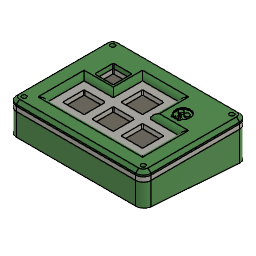
Hackpad (Autodesk Fusion 360 design; units mm, degrees)
Autodesk Fusion 360 part; units mm, degrees
sketch "Main" plane through (0, 0, 0) normal (0, 0, 1) x (1, 0, 0)
  line L0 (33.9, -23.9) -> (-33.9, -23.9)
  line L1 (-33.9, -23.9) -> (-33.9, 23.9)
  line L2 (-33.9, 23.9) -> (33.9, 23.9)
  line L3 (33.9, 23.9) -> (33.9, -23.9)
  line L4 (33.9, -23.9) -> (-33.9, 23.9) construction
  line L5 (-33.9, -23.9) -> (33.9, 23.9) construction
  line L6 (43.9, -33.9) -> (-43.9, -33.9)
  line L7 (-43.9, -33.9) -> (-43.9, 33.9)
  line L8 (-43.9, 33.9) -> (43.9, 33.9)
  line L9 (43.9, 33.9) -> (43.9, -33.9)
  circle A0 centre (-38.9, 28.9) radius 1.45
  circle A1 centre (-38.9, -28.9) radius 1.45
  circle A2 centre (38.9, 28.9) radius 1.45
  circle A3 centre (38.9, -28.9) radius 1.45
  arc A4 (-12.125, -3.025) -> (-12.625, -2.525) centre (-12.625, -3.025) ccw
  arc A5 (-12.625, -16.525) -> (-12.125, -16.025) centre (-12.625, -16.025) ccw
  line L10 (-25.625, -16.525) -> (-12.625, -16.525)
  arc A6 (-26.125, -16.025) -> (-25.625, -16.525) centre (-25.625, -16.025) ccw
  line L11 (-26.125, -3.025) -> (-26.125, -16.025)
  arc A7 (-25.625, -2.525) -> (-26.125, -3.025) centre (-25.625, -3.025) ccw
  line L12 (-25.625, -2.525) -> (-12.625, -2.525)
  line L13 (-6.575, -16.525) -> (6.425, -16.525)
  arc A8 (6.425, -16.525) -> (6.925, -16.025) centre (6.425, -16.025) ccw
  line L14 (6.925, -3.025) -> (6.925, -16.025)
  arc A9 (6.925, -3.025) -> (6.425, -2.525) centre (6.425, -3.025) ccw
  line L15 (-6.575, -2.525) -> (6.425, -2.525)
  arc A10 (-6.575, -2.525) -> (-7.075, -3.025) centre (-6.575, -3.025) ccw
  arc A11 (-7.075, -16.025) -> (-6.575, -16.525) centre (-6.575, -16.025) ccw
  line L16 (-7.075, -3.025) -> (-7.075, -16.025)
  line L17 (12.475, -16.525) -> (25.475, -16.525)
  arc A12 (25.475, -16.525) -> (25.975, -16.025) centre (25.475, -16.025) ccw
  line L18 (25.975, -3.025) -> (25.975, -16.025)
  arc A13 (25.975, -3.025) -> (25.475, -2.525) centre (25.475, -3.025) ccw
  line L19 (12.475, -2.525) -> (25.475, -2.525)
  arc A14 (12.475, -2.525) -> (11.975, -3.025) centre (12.475, -3.025) ccw
  arc A15 (11.975, -16.025) -> (12.475, -16.525) centre (12.475, -16.025) ccw
  arc A16 (6.425, 2.525) -> (6.925, 3.025) centre (6.425, 3.025) ccw
  arc A17 (-7.075, 3.025) -> (-6.575, 2.525) centre (-6.575, 3.025) ccw
  line L20 (-7.075, 16.025) -> (-7.075, 3.025)
  arc A18 (-6.575, 16.525) -> (-7.075, 16.025) centre (-6.575, 16.025) ccw
  line L21 (-6.575, 16.525) -> (6.425, 16.525)
  arc A19 (6.925, 16.025) -> (6.425, 16.525) centre (6.425, 16.025) ccw
  line L22 (6.925, 16.025) -> (6.925, 3.025)
  line L23 (-6.575, 2.525) -> (6.425, 2.525)
  line L24 (-31.175, 21.575) -> (31.025, 21.575)
  line L25 (-31.175, 21.575) -> (-31.175, -21.575)
  line L26 (-31.175, -21.575) -> (31.025, -21.575)
  line L27 (31.025, 21.575) -> (31.025, -21.575)
  line L28 (11.975, -3.025) -> (11.975, -16.025)
  line L29 (-12.125, -3.025) -> (-12.125, -16.025)
  line L30 (-12.125, 21.575) -> (-12.125, 2.525)
  line L31 (-31.175, 2.525) -> (-12.125, 2.525)
  line L32 (11.975, 2.525) -> (31.025, 2.525)
  line L33 (11.975, 21.575) -> (11.975, 2.525)
  line L34 (-16.95, 6.85) -> (-28.15, 6.85)
  line L35 (-28.65, 7.35) -> (-28.65, 18.55)
  line L36 (-28.15, 19.05) -> (-16.95, 19.05)
  line L37 (-16.45, 18.55) -> (-16.45, 7.35)
  line L38 (-16.45, 6.85) -> (-28.65, 19.05) construction
  line L39 (-28.65, 6.85) -> (-16.45, 19.05) construction
  arc A20 (-28.15, 19.05) -> (-28.65, 18.55) centre (-28.15, 18.55) ccw
  arc A21 (-16.45, 18.55) -> (-16.95, 19.05) centre (-16.95, 18.55) ccw
  arc A22 (-28.65, 7.35) -> (-28.15, 6.85) centre (-28.15, 7.35) ccw
  arc A23 (-16.95, 6.85) -> (-16.45, 7.35) centre (-16.95, 7.35) ccw
  line L40 (9.45, 0) -> (-9.6, 0)
  line L41 (-9.6, 0) -> (-9.6, 19.05)
  line L42 (-9.6, 19.05) -> (9.45, 19.05)
  line L43 (9.45, 19.05) -> (9.45, 0)
  line L44 (9.45, 0) -> (-9.6, 19.05) construction
  line L45 (-9.6, 0) -> (9.45, 19.05) construction
  line L46 (-9.6, -19.05) -> (-28.65, -19.05)
  line L47 (-28.65, -19.05) -> (-28.65, 0)
  line L48 (-28.65, 0) -> (-9.6, 0)
  line L49 (-9.6, 0) -> (-9.6, -19.05)
  line L50 (0, 23.9) -> (0, -33.9) construction
  arc A24 (16.95, 19.05) -> (16.45, 18.55) centre (16.95, 18.55) ccw
  line L51 (16.45, 18.55) -> (16.45, 7.35)
  arc A25 (16.45, 7.35) -> (16.95, 6.85) centre (16.95, 7.35) ccw
  line L52 (16.95, 6.85) -> (28.15, 6.85)
  arc A26 (28.15, 6.85) -> (28.65, 7.35) centre (28.15, 7.35) ccw
  line L53 (28.65, 7.35) -> (28.65, 18.55)
  arc A27 (28.65, 18.55) -> (28.15, 19.05) centre (28.15, 18.55) ccw
  line L54 (28.15, 19.05) -> (16.95, 19.05)
  spline S0 degree 3 poles (22.2716, 17.9984) (22.4772, 17.9984) (22.6828, 17.9984) (22.8884, 17.9984) knots 0 0 0 0 1 1 1 1
  spline S1 degree 3 poles (22.8884, 17.9984) (22.9326, 17.9794) (23.084, 17.9645) (23.1108, 17.9887) knots 0 0 0 0 1 1 1 1
  spline S2 degree 3 poles (23.1108, 17.9887) (23.1434, 17.9593) (23.3545, 17.9395) (23.4085, 17.9401) knots 0 0 0 0 1 1 1 1
  spline S3 degree 3 poles (23.4085, 17.9401) (23.4406, 17.9405) (23.4795, 17.918) (23.5093, 17.9135) knots 0 0 0 0 1 1 1 1
  spline S4 degree 3 poles (23.5093, 17.9135) (23.5998, 17.8996) (23.701, 17.8877) (23.795, 17.8676) knots 0 0 0 0 1 1 1 1
  spline S5 degree 3 poles (23.795, 17.8676) (23.8778, 17.85) (23.9581, 17.8109) (24.0419, 17.7948) knots 0 0 0 0 1 1 1 1
  spline S6 degree 3 poles (24.0419, 17.7948) (24.058, 17.7918) (24.0679, 17.7758) (24.0836, 17.7722) knots 0 0 0 0 1 1 1 1
  spline S7 degree 3 poles (24.0836, 17.7722) (24.2356, 17.7361) (24.382, 17.6718) (24.5308, 17.6218) knots 0 0 0 0 1 1 1 1
  spline S8 degree 3 poles (24.5308, 17.6218) (24.5703, 17.6085) (24.6731, 17.5303) (24.6983, 17.5523) knots 0 0 0 0 1 1 1 1
  spline S9 degree 3 poles (24.6983, 17.5523) (24.7382, 17.498) (24.8225, 17.4853) (24.8785, 17.4541) knots 0 0 0 0 1 1 1 1
  spline S10 degree 3 poles (24.8785, 17.4541) (24.9607, 17.4083) (25.0549, 17.3585) (25.1345, 17.3031) knots 0 0 0 0 1 1 1 1
  spline S11 degree 3 poles (25.1345, 17.3031) (25.4383, 17.0916) (25.751, 16.8719) (25.9987, 16.579) knots 0 0 0 0 1 1 1 1
  spline S12 degree 3 poles (25.9987, 16.579) (26.1039, 16.4548) (26.216, 16.3169) (26.3112, 16.1875) knots 0 0 0 0 1 1 1 1
  spline S13 degree 3 poles (26.3112, 16.1875) (26.3854, 16.0869) (26.442, 15.9672) (26.5144, 15.8634) knots 0 0 0 0 1 1 1 1
  spline S14 degree 3 poles (26.5144, 15.8634) (26.567, 15.7884) (26.6319, 15.5622) (26.6964, 15.5146) knots 0 0 0 0 1 1 1 1
  spline S15 degree 3 poles (26.6964, 15.5146) (26.6815, 15.4925) (26.715, 15.4554) (26.7295, 15.4265) knots 0 0 0 0 1 1 1 1
  spline S16 degree 3 poles (26.7295, 15.4265) (26.751, 15.3836) (26.8186, 15.2094) (26.8289, 15.1655) knots 0 0 0 0 1 1 1 1
  spline S17 degree 3 poles (26.8289, 15.1655) (26.8895, 14.9066) (27.0063, 14.6397) (27.0157, 14.3835) knots 0 0 0 0 1 1 1 1
  spline S18 degree 3 poles (27.0157, 14.3835) (27.0165, 14.3601) (27.0395, 14.3357) (27.0419, 14.3136) knots 0 0 0 0 1 1 1 1
  spline S19 degree 3 poles (27.0419, 14.3136) (27.0494, 14.2414) (27.05, 14.1612) (27.0554, 14.0957) knots 0 0 0 0 1 1 1 1
  spline S20 degree 3 poles (27.0554, 14.0957) (27.0579, 14.0646) (27.0812, 14.0261) (27.0845, 13.9961) knots 0 0 0 0 1 1 1 1
  spline S21 degree 3 poles (27.0845, 13.9961) (27.0893, 13.9552) (27.0613, 13.9424) (27.0935, 13.9072) knots 0 0 0 0 1 1 1 1
  spline S22 degree 3 poles (27.0935, 13.9072) (27.0431, 13.8523) (27.1145, 13.7201) (27.1062, 13.6592) knots 0 0 0 0 1 1 1 1
  spline S23 degree 3 poles (27.1062, 13.6592) (27.0869, 13.5175) (27.0736, 13.1639) (27.0945, 13.0242) knots 0 0 0 0 1 1 1 1
  spline S24 degree 3 poles (27.0945, 13.0242) (27.0996, 12.9893) (27.1085, 12.9617) (27.1072, 12.925) knots 0 0 0 0 1 1 1 1
  spline S25 degree 3 poles (27.1072, 12.925) (27.106, 12.8912) (27.0897, 12.8686) (27.0883, 12.8357) knots 0 0 0 0 1 1 1 1
  spline S26 degree 3 poles (27.0883, 12.8357) (27.0855, 12.7708) (27.0597, 12.5648) (27.0935, 12.5281) knots 0 0 0 0 1 1 1 1
  spline S27 degree 3 poles (27.0935, 12.5281) (27.0613, 12.4858) (27.0871, 12.4636) (27.0861, 12.4189) knots 0 0 0 0 1 1 1 1
  spline S28 degree 3 poles (27.0861, 12.4189) (27.0849, 12.361) (27.0294, 12.2788) (27.0734, 12.2304) knots 0 0 0 0 1 1 1 1
  spline S29 degree 3 poles (27.0734, 12.2304) (27.0415, 12.1953) (27.0439, 12.1016) (27.0444, 12.0518) knots 0 0 0 0 1 1 1 1
  spline S30 degree 3 poles (27.0444, 12.0518) (27.0448, 12.0125) (27.0167, 11.9735) (27.0157, 11.9328) knots 0 0 0 0 1 1 1 1
  spline S31 degree 3 poles (27.0157, 11.9328) (27.0141, 11.8609) (27.0046, 11.771) (26.9887, 11.6964) knots 0 0 0 0 1 1 1 1
  spline S32 degree 3 poles (26.9887, 11.6964) (26.9837, 11.674) (26.9623, 11.6478) (26.9577, 11.6234) knots 0 0 0 0 1 1 1 1
  spline S33 degree 3 poles (26.9577, 11.6234) (26.9111, 11.3785) (26.8113, 11.1164) (26.6883, 10.9025) knots 0 0 0 0 1 1 1 1
  spline S34 degree 3 poles (26.6883, 10.9025) (26.5359, 10.638) (26.217, 10.3324) (25.959, 10.1774) knots 0 0 0 0 1 1 1 1
  spline S35 degree 3 poles (25.959, 10.1774) (25.8709, 10.1246) (25.7862, 10.0796) (25.6921, 10.0333) knots 0 0 0 0 1 1 1 1
  spline S36 degree 3 poles (25.6921, 10.0333) (25.6417, 10.0087) (25.5661, 10.0024) (25.5318, 9.9544) knots 0 0 0 0 1 1 1 1
  spline S37 degree 3 poles (25.5318, 9.9544) (25.527, 9.9575) (25.529, 9.9669) (25.5218, 9.968) knots 0 0 0 0 1 1 1 1
  spline S38 degree 3 poles (25.5218, 9.968) (25.5197, 9.9684) (25.5038, 9.9522) (25.5004, 9.95) knots 0 0 0 0 1 1 1 1
  spline S39 degree 3 poles (25.5004, 9.95) (25.4738, 9.9327) (25.4397, 9.9355) (25.4127, 9.9236) knots 0 0 0 0 1 1 1 1
  spline S40 degree 3 poles (25.4127, 9.9236) (25.3724, 9.8541) (25.4006, 9.5845) (25.4006, 9.492) knots 0 0 0 0 1 1 1 1
  spline S41 degree 3 poles (25.4006, 9.492) (25.4006, 9.1666) (25.451, 8.6266) (25.3405, 8.3498) knots 0 0 0 0 1 1 1 1
  spline S42 degree 3 poles (25.3405, 8.3498) (25.27, 8.1732) (25.1008, 8.0081) (24.9275, 7.9172) knots 0 0 0 0 1 1 1 1
  spline S43 degree 3 poles (24.9275, 7.9172) (24.8791, 7.892) (24.7993, 7.8638) (24.7475, 7.8531) knots 0 0 0 0 1 1 1 1
  spline S44 degree 3 poles (24.7475, 7.8531) (24.7194, 7.8471) (24.7027, 7.859) (24.6749, 7.8416) knots 0 0 0 0 1 1 1 1
  spline S45 degree 3 poles (24.6749, 7.8416) (24.5949, 7.8416) (24.5148, 7.8416) (24.4346, 7.8416) knots 0 0 0 0 1 1 1 1
  spline S46 degree 3 poles (24.4346, 7.8416) (24.4056, 7.861) (24.3828, 7.8473) (24.3528, 7.8559) knots 0 0 0 0 1 1 1 1
  spline S47 degree 3 poles (24.3528, 7.8559) (24.2677, 7.8803) (24.1572, 7.9281) (24.0824, 7.9737) knots 0 0 0 0 1 1 1 1
  spline S48 degree 3 poles (24.0824, 7.9737) (24.0443, 7.997) (24.0078, 8.0718) (23.9641, 8.0652) knots 0 0 0 0 1 1 1 1
  spline S49 degree 3 poles (23.9641, 8.0652) (23.9417, 8.1222) (23.8843, 8.1631) (23.8448, 8.2111) knots 0 0 0 0 1 1 1 1
  spline S50 degree 3 poles (23.8448, 8.2111) (23.8181, 8.2434) (23.7587, 8.3702) (23.7484, 8.4123) knots 0 0 0 0 1 1 1 1
  spline S51 degree 3 poles (23.7484, 8.4123) (23.6914, 8.6421) (23.7095, 8.9066) (23.7095, 9.1546) knots 0 0 0 0 1 1 1 1
  spline S52 degree 3 poles (23.7095, 9.1546) (23.7095, 9.2572) (23.7095, 9.3596) (23.7095, 9.4622) knots 0 0 0 0 1 1 1 1
  spline S53 degree 3 poles (23.7095, 9.4622) (23.7095, 9.5015) (23.723, 9.5543) (23.6863, 9.5763) knots 0 0 0 0 1 1 1 1
  spline S54 degree 3 poles (23.6863, 9.5763) (23.6464, 9.573) (23.6369, 9.573) (23.597, 9.5763) knots 0 0 0 0 1 1 1 1
  spline S55 degree 3 poles (23.597, 9.5763) (23.544, 9.5698) (23.4912, 9.563) (23.4382, 9.5565) knots 0 0 0 0 1 1 1 1
  spline S56 degree 3 poles (23.4382, 9.5565) (23.4613, 9.4164) (23.4418, 9.2574) (23.4418, 9.115) knots 0 0 0 0 1 1 1 1
  spline S57 degree 3 poles (23.4418, 9.115) (23.4418, 8.7514) (23.4509, 8.4607) (23.2527, 8.1635) knots 0 0 0 0 1 1 1 1
  spline S58 degree 3 poles (23.2527, 8.1635) (23.2092, 8.0984) (23.0898, 7.992) (23.0221, 7.9555) knots 0 0 0 0 1 1 1 1
  spline S59 degree 3 poles (23.0221, 7.9555) (22.9693, 7.9267) (22.8959, 7.9128) (22.8529, 7.8708) knots 0 0 0 0 1 1 1 1
  spline S60 degree 3 poles (22.8529, 7.8708) (22.8306, 7.8878) (22.7316, 7.8624) (22.7003, 7.8416) knots 0 0 0 0 1 1 1 1
  spline S61 degree 3 poles (22.7003, 7.8416) (22.6201, 7.8416) (22.5399, 7.8416) (22.4597, 7.8416) knots 0 0 0 0 1 1 1 1
  spline S62 degree 3 poles (22.4597, 7.8416) (22.4151, 7.8718) (22.3671, 7.8596) (22.3189, 7.8761) knots 0 0 0 0 1 1 1 1
  spline S63 degree 3 poles (22.3189, 7.8761) (22.2298, 7.9067) (22.0371, 8.0047) (21.9744, 8.0823) knots 0 0 0 0 1 1 1 1
  spline S64 degree 3 poles (21.9744, 8.0823) (21.7025, 8.4184) (21.7182, 8.6715) (21.7182, 9.105) knots 0 0 0 0 1 1 1 1
  spline S65 degree 3 poles (21.7182, 9.105) (21.7182, 9.2505) (21.6983, 9.4132) (21.7218, 9.5565) knots 0 0 0 0 1 1 1 1
  spline S66 degree 3 poles (21.7218, 9.5565) (21.6688, 9.563) (21.616, 9.5698) (21.563, 9.5763) knots 0 0 0 0 1 1 1 1
  spline S67 degree 3 poles (21.563, 9.5763) (21.5231, 9.573) (21.5136, 9.573) (21.4737, 9.5763) knots 0 0 0 0 1 1 1 1
  spline S68 degree 3 poles (21.4737, 9.5763) (21.4275, 9.5485) (21.4505, 9.4237) (21.4505, 9.3729) knots 0 0 0 0 1 1 1 1
  spline S69 degree 3 poles (21.4505, 9.3729) (21.4505, 9.1745) (21.4505, 8.9761) (21.4505, 8.7776) knots 0 0 0 0 1 1 1 1
  spline S70 degree 3 poles (21.4505, 8.7776) (21.4505, 8.6284) (21.4432, 8.4766) (21.3824, 8.3434) knots 0 0 0 0 1 1 1 1
  spline S71 degree 3 poles (21.3824, 8.3434) (21.3654, 8.3059) (21.3412, 8.2404) (21.3154, 8.2111) knots 0 0 0 0 1 1 1 1
  spline S72 degree 3 poles (21.3154, 8.2111) (21.3017, 8.1954) (21.2384, 8.1488) (21.2368, 8.1273) knots 0 0 0 0 1 1 1 1
  spline S73 degree 3 poles (21.2368, 8.1273) (21.2362, 8.122) (21.2427, 8.1182) (21.2435, 8.1129) knots 0 0 0 0 1 1 1 1
  spline S74 degree 3 poles (21.2435, 8.1129) (21.1782, 8.088) (21.1368, 8.012) (21.0776, 7.9734) knots 0 0 0 0 1 1 1 1
  spline S75 degree 3 poles (21.0776, 7.9734) (21.0165, 7.9335) (20.8766, 7.8688) (20.8072, 7.8559) knots 0 0 0 0 1 1 1 1
  spline S76 degree 3 poles (20.8072, 7.8559) (20.776, 7.8501) (20.7538, 7.8612) (20.7252, 7.8416) knots 0 0 0 0 1 1 1 1
  spline S77 degree 3 poles (20.7252, 7.8416) (20.645, 7.8416) (20.5651, 7.8416) (20.4849, 7.8416) knots 0 0 0 0 1 1 1 1
  spline S78 degree 3 poles (20.4849, 7.8416) (20.4399, 7.8684) (20.3827, 7.8622) (20.3345, 7.8779) knots 0 0 0 0 1 1 1 1
  spline S79 degree 3 poles (20.3345, 7.8779) (20.1944, 7.9229) (20.0555, 8.0232) (19.9576, 8.1325) knots 0 0 0 0 1 1 1 1
  spline S80 degree 3 poles (19.9576, 8.1325) (19.8876, 8.2107) (19.8301, 8.3172) (19.7943, 8.4109) knots 0 0 0 0 1 1 1 1
  spline S81 degree 3 poles (19.7943, 8.4109) (19.7469, 8.5349) (19.7594, 8.6879) (19.7594, 8.8272) knots 0 0 0 0 1 1 1 1
  spline S82 degree 3 poles (19.7594, 8.8272) (19.7594, 9.0654) (19.7594, 9.3035) (19.7594, 9.5416) knots 0 0 0 0 1 1 1 1
  spline S83 degree 3 poles (19.7594, 9.5416) (19.7594, 9.6559) (19.7862, 9.8101) (19.7523, 9.9186) knots 0 0 0 0 1 1 1 1
  spline S84 degree 3 poles (19.7523, 9.9186) (19.7288, 9.9353) (19.6453, 9.9665) (19.6282, 9.9544) knots 0 0 0 0 1 1 1 1
  spline S85 degree 3 poles (19.6282, 9.9544) (19.5953, 9.9986) (19.3961, 10.0689) (19.3391, 10.098) knots 0 0 0 0 1 1 1 1
  spline S86 degree 3 poles (19.3391, 10.098) (19.1699, 10.1849) (19.0292, 10.309) (18.8754, 10.4217) knots 0 0 0 0 1 1 1 1
  spline S87 degree 3 poles (18.8754, 10.4217) (18.748, 10.5151) (18.5432, 10.7767) (18.4688, 10.9102) knots 0 0 0 0 1 1 1 1
  spline S88 degree 3 poles (18.4688, 10.9102) (18.4336, 10.9729) (18.4073, 11.0938) (18.3447, 11.139) knots 0 0 0 0 1 1 1 1
  spline S89 degree 3 poles (18.3447, 11.139) (18.365, 11.1696) (18.3027, 11.2454) (18.2914, 11.2896) knots 0 0 0 0 1 1 1 1
  spline S90 degree 3 poles (18.2914, 11.2896) (18.2682, 11.3799) (18.214, 11.4984) (18.2013, 11.5873) knots 0 0 0 0 1 1 1 1
  spline S91 degree 3 poles (18.2013, 11.5873) (18.1925, 11.647) (18.1798, 11.7504) (18.1463, 11.7939) knots 0 0 0 0 1 1 1 1
  spline S92 degree 3 poles (18.1463, 11.7939) (18.1781, 11.8292) (18.1348, 11.8687) (18.1354, 11.9129) knots 0 0 0 0 1 1 1 1
  spline S93 degree 3 poles (18.1354, 11.9129) (18.136, 11.9663) (18.115, 12.1993) (18.0864, 12.2304) knots 0 0 0 0 1 1 1 1
  spline S94 degree 3 poles (18.0864, 12.2304) (18.1277, 12.2755) (18.0804, 12.3543) (18.0751, 12.409) knots 0 0 0 0 1 1 1 1
  spline S95 degree 3 poles (18.0751, 12.409) (18.0709, 12.4539) (18.1017, 12.4797) (18.0667, 12.5182) knots 0 0 0 0 1 1 1 1
  spline S96 degree 3 poles (18.0667, 12.5182) (18.1042, 12.5592) (18.0707, 12.8236) (18.0548, 12.8853) knots 0 0 0 0 1 1 1 1
  spline S97 degree 3 poles (18.0548, 12.8853) (18.0392, 12.9468) (18.0655, 13.0202) (18.0655, 13.0837) knots 0 0 0 0 1 1 1 1
  spline S98 degree 3 poles (18.0655, 13.0837) (18.0655, 13.2621) (18.0743, 13.4447) (18.0528, 13.6195) knots 0 0 0 0 1 1 1 1
  spline S99 degree 3 poles (18.0528, 13.6195) (18.0437, 13.6939) (18.1191, 13.8695) (18.0667, 13.9271) knots 0 0 0 0 1 1 1 1
  spline S100 degree 3 poles (18.0667, 13.9271) (18.0973, 13.9606) (18.1122, 14.2434) (18.1219, 14.3126) knots 0 0 0 0 1 1 1 1
  spline S101 degree 3 poles (18.1219, 14.3126) (18.1348, 14.4061) (18.1521, 14.5004) (18.1683, 14.5914) knots 0 0 0 0 1 1 1 1
  spline S102 degree 3 poles (18.1683, 14.5914) (18.1737, 14.6214) (18.1989, 14.6506) (18.2041, 14.6815) knots 0 0 0 0 1 1 1 1
  spline S103 degree 3 poles (18.2041, 14.6815) (18.2138, 14.7379) (18.2175, 14.7921) (18.2324, 14.848) knots 0 0 0 0 1 1 1 1
  spline S104 degree 3 poles (18.2324, 14.848) (18.2614, 14.9558) (18.3064, 15.0578) (18.3309, 15.1655) knots 0 0 0 0 1 1 1 1
  spline S105 degree 3 poles (18.3309, 15.1655) (18.3424, 15.2163) (18.4055, 15.3774) (18.4303, 15.4267) knots 0 0 0 0 1 1 1 1
  spline S106 degree 3 poles (18.4303, 15.4267) (18.445, 15.4552) (18.4781, 15.4927) (18.4636, 15.5146) knots 0 0 0 0 1 1 1 1
  spline S107 degree 3 poles (18.4636, 15.5146) (18.5305, 15.5666) (18.5626, 15.7277) (18.6158, 15.8019) knots 0 0 0 0 1 1 1 1
  spline S108 degree 3 poles (18.6158, 15.8019) (18.6704, 15.8783) (18.7029, 15.9865) (18.765, 16.0613) knots 0 0 0 0 1 1 1 1
  spline S109 degree 3 poles (18.765, 16.0613) (18.8252, 16.1335) (18.8821, 16.2176) (18.9309, 16.2968) knots 0 0 0 0 1 1 1 1
  spline S110 degree 3 poles (18.9309, 16.2968) (18.9722, 16.3639) (19.0413, 16.4391) (19.0917, 16.4996) knots 0 0 0 0 1 1 1 1
  spline S111 degree 3 poles (19.0917, 16.4996) (19.1038, 16.5141) (19.1264, 16.5195) (19.1371, 16.5365) knots 0 0 0 0 1 1 1 1
  spline S112 degree 3 poles (19.1371, 16.5365) (19.2133, 16.657) (19.348, 16.775) (19.4627, 16.8655) knots 0 0 0 0 1 1 1 1
  spline S113 degree 3 poles (19.4627, 16.8655) (19.5522, 16.9362) (19.6201, 17.0211) (19.7094, 17.0848) knots 0 0 0 0 1 1 1 1
  spline S114 degree 3 poles (19.7094, 17.0848) (19.8493, 17.1844) (19.9956, 17.2682) (20.1327, 17.3708) knots 0 0 0 0 1 1 1 1
  spline S115 degree 3 poles (20.1327, 17.3708) (20.1468, 17.3815) (20.1662, 17.3793) (20.1811, 17.3866) knots 0 0 0 0 1 1 1 1
  spline S116 degree 3 poles (20.1811, 17.3866) (20.2013, 17.3966) (20.214, 17.419) (20.2323, 17.4287) knots 0 0 0 0 1 1 1 1
  spline S117 degree 3 poles (20.2323, 17.4287) (20.2833, 17.4557) (20.3468, 17.4775) (20.4004, 17.5057) knots 0 0 0 0 1 1 1 1
  spline S118 degree 3 poles (20.4004, 17.5057) (20.6157, 17.6188) (20.8441, 17.7091) (21.085, 17.7742) knots 0 0 0 0 1 1 1 1
  spline S119 degree 3 poles (21.085, 17.7742) (21.1487, 17.7914) (21.2114, 17.8339) (21.2771, 17.8448) knots 0 0 0 0 1 1 1 1
  spline S120 degree 3 poles (21.2771, 17.8448) (21.3412, 17.8555) (21.4047, 17.8672) (21.4656, 17.8847) knots 0 0 0 0 1 1 1 1
  spline S121 degree 3 poles (21.4656, 17.8847) (21.5511, 17.9091) (21.6878, 17.9296) (21.7714, 17.9311) knots 0 0 0 0 1 1 1 1
  spline S122 degree 3 poles (21.7714, 17.9311) (21.8065, 17.9319) (21.846, 17.9605) (21.8805, 17.9599) knots 0 0 0 0 1 1 1 1
  spline S123 degree 3 poles (21.8805, 17.9599) (21.9313, 17.9589) (22.0297, 17.9532) (22.069, 17.9891) knots 0 0 0 0 1 1 1 1
  spline S124 degree 3 poles (22.069, 17.9891) (22.0982, 17.9623) (22.2248, 17.9784) (22.2716, 17.9984) knots 0 0 0 0 1 1 1 1
  spline S125 degree 3 poles (20.474, 15.4554) (20.2771, 15.435) (20.0807, 15.3765) (19.909, 15.2776) knots 0 0 0 0 1 1 1 1
  spline S126 degree 3 poles (19.909, 15.2776) (19.0863, 14.8038) (18.9414, 13.6485) (19.6542, 13.0053) knots 0 0 0 0 1 1 1 1
  spline S127 degree 3 poles (19.6542, 13.0053) (19.7991, 12.8748) (19.9656, 12.7799) (20.1483, 12.7156) knots 0 0 0 0 1 1 1 1
  spline S128 degree 3 poles (20.1483, 12.7156) (20.3432, 12.6469) (20.5526, 12.6251) (20.7591, 12.6452) knots 0 0 0 0 1 1 1 1
  spline S129 degree 3 poles (20.7591, 12.6452) (20.9296, 12.6614) (21.1003, 12.7158) (21.2507, 12.7952) knots 0 0 0 0 1 1 1 1
  spline S130 degree 3 poles (21.2507, 12.7952) (22.1258, 13.2571) (22.2855, 14.4625) (21.5273, 15.1165) knots 0 0 0 0 1 1 1 1
  spline S131 degree 3 poles (21.5273, 15.1165) (21.386, 15.2381) (21.2267, 15.3247) (21.052, 15.386) knots 0 0 0 0 1 1 1 1
  spline S132 degree 3 poles (21.052, 15.386) (20.8705, 15.4497) (20.6665, 15.4755) (20.474, 15.4554) knots 0 0 0 0 1 1 1 1
  spline S133 degree 3 poles (24.4233, 15.4554) (24.226, 15.4342) (24.0308, 15.3759) (23.8589, 15.2768) knots 0 0 0 0 1 1 1 1
  spline S134 degree 3 poles (23.8589, 15.2768) (23.0535, 14.8129) (22.8997, 13.703) (23.5635, 13.0452) knots 0 0 0 0 1 1 1 1
  spline S135 degree 3 poles (23.5635, 13.0452) (23.7153, 12.8948) (23.898, 12.7874) (24.0973, 12.7156) knots 0 0 0 0 1 1 1 1
  spline S136 degree 3 poles (24.0973, 12.7156) (24.2909, 12.6458) (24.5027, 12.6259) (24.7082, 12.6448) knots 0 0 0 0 1 1 1 1
  spline S137 degree 3 poles (24.7082, 12.6448) (25.5316, 12.7212) (26.1356, 13.576) (25.9288, 14.3795) knots 0 0 0 0 1 1 1 1
  spline S138 degree 3 poles (25.9288, 14.3795) (25.806, 14.8564) (25.4625, 15.2213) (25.0017, 15.3866) knots 0 0 0 0 1 1 1 1
  spline S139 degree 3 poles (25.0017, 15.3866) (24.8217, 15.4513) (24.6146, 15.4759) (24.4233, 15.4554) knots 0 0 0 0 1 1 1 1
  spline S140 degree 3 poles (22.6048, 10.941) (22.6737, 10.8263) (22.7389, 10.7245) (22.8755, 10.6816) knots 0 0 0 0 1 1 1 1
  spline S141 degree 3 poles (22.8755, 10.6816) (23.1396, 10.5987) (23.4009, 10.792) (23.4261, 11.0596) knots 0 0 0 0 1 1 1 1
  spline S142 degree 3 poles (23.4261, 11.0596) (23.4394, 11.2019) (23.3609, 11.347) (23.2473, 11.4291) knots 0 0 0 0 1 1 1 1
  spline S143 degree 3 poles (23.2473, 11.4291) (23.2098, 11.4563) (23.1575, 11.4643) (23.1227, 11.4928) knots 0 0 0 0 1 1 1 1
  spline S144 degree 3 poles (23.1227, 11.4928) (23.0761, 11.5311) (23.0543, 11.6018) (23.0053, 11.6438) knots 0 0 0 0 1 1 1 1
  spline S145 degree 3 poles (23.0053, 11.6438) (22.8646, 11.7645) (22.6677, 11.8068) (22.4861, 11.7861) knots 0 0 0 0 1 1 1 1
  spline S146 degree 3 poles (22.4861, 11.7861) (22.3587, 11.7714) (22.2194, 11.7127) (22.129, 11.6198) knots 0 0 0 0 1 1 1 1
  spline S147 degree 3 poles (22.129, 11.6198) (22.0932, 11.5829) (22.0744, 11.525) (22.0375, 11.4926) knots 0 0 0 0 1 1 1 1
  spline S148 degree 3 poles (22.0375, 11.4926) (22.0025, 11.4619) (21.946, 11.4535) (21.9071, 11.4246) knots 0 0 0 0 1 1 1 1
  spline S149 degree 3 poles (21.9071, 11.4246) (21.7652, 11.3188) (21.7003, 11.1343) (21.7503, 10.963) knots 0 0 0 0 1 1 1 1
  spline S150 degree 3 poles (21.7503, 10.963) (21.8226, 10.7167) (22.1051, 10.6017) (22.3339, 10.7017) knots 0 0 0 0 1 1 1 1
  spline S151 degree 3 poles (22.3339, 10.7017) (22.4451, 10.7503) (22.4967, 10.8434) (22.5552, 10.941) knots 0 0 0 0 1 1 1 1
  spline S152 degree 3 poles (22.5552, 10.941) (22.5717, 10.941) (22.5883, 10.941) (22.6048, 10.941) knots 0 0 0 0 1 1 1 1
  spline S153 degree 3 poles (20.474, 15.4554) (20.6665, 15.4755) (20.8705, 15.4497) (21.052, 15.386) knots 0 0 0 0 1 1 1 1
  spline S154 degree 3 poles (21.052, 15.386) (21.2267, 15.3247) (21.386, 15.2381) (21.5273, 15.1165) knots 0 0 0 0 1 1 1 1
  spline S155 degree 3 poles (21.5273, 15.1165) (22.2855, 14.4625) (22.1258, 13.2571) (21.2507, 12.7952) knots 0 0 0 0 1 1 1 1
  spline S156 degree 3 poles (21.2507, 12.7952) (21.1003, 12.7158) (20.9296, 12.6614) (20.7591, 12.6452) knots 0 0 0 0 1 1 1 1
  spline S157 degree 3 poles (20.7591, 12.6452) (20.5526, 12.6251) (20.3432, 12.6469) (20.1483, 12.7156) knots 0 0 0 0 1 1 1 1
  spline S158 degree 3 poles (20.1483, 12.7156) (19.9656, 12.7799) (19.7991, 12.8748) (19.6542, 13.0053) knots 0 0 0 0 1 1 1 1
  spline S159 degree 3 poles (19.6542, 13.0053) (18.9414, 13.6485) (19.0863, 14.8038) (19.909, 15.2776) knots 0 0 0 0 1 1 1 1
  spline S160 degree 3 poles (19.909, 15.2776) (20.0807, 15.3765) (20.2771, 15.435) (20.474, 15.4554) knots 0 0 0 0 1 1 1 1
  spline S161 degree 3 poles (24.4233, 15.4554) (24.6146, 15.4759) (24.8217, 15.4513) (25.0017, 15.3866) knots 0 0 0 0 1 1 1 1
  spline S162 degree 3 poles (25.0017, 15.3866) (25.4625, 15.2213) (25.806, 14.8564) (25.9288, 14.3795) knots 0 0 0 0 1 1 1 1
  spline S163 degree 3 poles (25.9288, 14.3795) (26.1356, 13.576) (25.5316, 12.7212) (24.7082, 12.6448) knots 0 0 0 0 1 1 1 1
  spline S164 degree 3 poles (24.7082, 12.6448) (24.5027, 12.6259) (24.2909, 12.6458) (24.0973, 12.7156) knots 0 0 0 0 1 1 1 1
  spline S165 degree 3 poles (24.0973, 12.7156) (23.898, 12.7874) (23.7153, 12.8948) (23.5635, 13.0452) knots 0 0 0 0 1 1 1 1
  spline S166 degree 3 poles (23.5635, 13.0452) (22.8997, 13.703) (23.0535, 14.8129) (23.8589, 15.2768) knots 0 0 0 0 1 1 1 1
  spline S167 degree 3 poles (23.8589, 15.2768) (24.0308, 15.3759) (24.226, 15.4342) (24.4233, 15.4554) knots 0 0 0 0 1 1 1 1
  spline S168 degree 3 poles (22.6048, 10.941) (22.5883, 10.941) (22.5717, 10.941) (22.5552, 10.941) knots 0 0 0 0 1 1 1 1
  spline S169 degree 3 poles (22.5552, 10.941) (22.4967, 10.8434) (22.4451, 10.7503) (22.3339, 10.7017) knots 0 0 0 0 1 1 1 1
  spline S170 degree 3 poles (22.3339, 10.7017) (22.1051, 10.6017) (21.8226, 10.7167) (21.7503, 10.963) knots 0 0 0 0 1 1 1 1
  spline S171 degree 3 poles (21.7503, 10.963) (21.7003, 11.1343) (21.7652, 11.3188) (21.9071, 11.4246) knots 0 0 0 0 1 1 1 1
  spline S172 degree 3 poles (21.9071, 11.4246) (21.946, 11.4535) (22.0025, 11.4619) (22.0375, 11.4926) knots 0 0 0 0 1 1 1 1
  spline S173 degree 3 poles (22.0375, 11.4926) (22.0744, 11.525) (22.0932, 11.5829) (22.129, 11.6198) knots 0 0 0 0 1 1 1 1
  spline S174 degree 3 poles (22.129, 11.6198) (22.2194, 11.7127) (22.3587, 11.7714) (22.4861, 11.7861) knots 0 0 0 0 1 1 1 1
  spline S175 degree 3 poles (22.4861, 11.7861) (22.6677, 11.8068) (22.8646, 11.7645) (23.0053, 11.6438) knots 0 0 0 0 1 1 1 1
  spline S176 degree 3 poles (23.0053, 11.6438) (23.0543, 11.6018) (23.0761, 11.5311) (23.1227, 11.4928) knots 0 0 0 0 1 1 1 1
  spline S177 degree 3 poles (23.1227, 11.4928) (23.1575, 11.4643) (23.2098, 11.4563) (23.2473, 11.4291) knots 0 0 0 0 1 1 1 1
  spline S178 degree 3 poles (23.2473, 11.4291) (23.3609, 11.347) (23.4394, 11.2019) (23.4261, 11.0596) knots 0 0 0 0 1 1 1 1
  spline S179 degree 3 poles (23.4261, 11.0596) (23.4009, 10.792) (23.1396, 10.5987) (22.8755, 10.6816) knots 0 0 0 0 1 1 1 1
  spline S180 degree 3 poles (22.8755, 10.6816) (22.7389, 10.7245) (22.6737, 10.8263) (22.6048, 10.941) knots 0 0 0 0 1 1 1 1
  point P0 (-38.9, 28.9)
  point P1 (-22.55, 12.95)
  point P2 (-0.075, 9.525)
  dimension "d1" = 67.8
  dimension "d2" = 47.8
  dimension "d3" = -10
  dimension "d4" = 2.9
  dimension "d5" = 5
  dimension "d6" = 5
  dimension "d7" = 2.9
  dimension "d8" = 2.9
  dimension "d9" = 2.9
  dimension "d10" = 5
  dimension "d11" = 5
  dimension "d12" = 5
  dimension "d13" = 5
  dimension "d14" = 5
  dimension "d15" = 5
  dimension "d18" = 87.8
  dimension "d37" = 5.05
  dimension "d38" = 5.05
  dimension "d39" = 5.05
  dimension "d40" = 5.05
  dimension "d41" = 5.05
  dimension "d42" = 5.05
  dimension "d43" = 5.05
  dimension "d44" = 5.05
  dimension "d71" = 12.2
  dimension "d72" = 12.2
  dimension "d73" = 0.5
  dimension "d74" = 0.5
  dimension "d75" = 0.5
  dimension "d76" = 0.5
  dimension "d79" = 62.2
  dimension "d80" = 19.05
  dimension "d81" = 19.05
  dimension "d82" = 7
  dimension "d83" = 7
  dimension "d84" = 19.05
  dimension "d85" = 19.05
  dimension "d86" = 2.525
  dimension "d87" = 2.525
  constraint horizontal L0
  constraint perpendicular L0 L1
  constraint parallel L0 L2
  constraint parallel L1 L3
  constraint coincident L4 origin
  constraint coincident L5 origin
  constraint tangent A4 L29
  constraint tangent A14 L28
  constraint tangent A17 L23
  constraint perpendicular L1 L26
  constraint perpendicular L24 L30
  constraint parallel L12 L31
  constraint coincident L25 L31.start
  constraint coincident L24 L30.start
  constraint perpendicular L22 L32
  constraint parallel L22 L33
  constraint coincident L24 L33.start
  constraint coincident L27 L32.end
  constraint horizontal L34
  constraint perpendicular L34 L35
  constraint parallel L34 L36
  constraint parallel L35 L37
  constraint coincident L38 P1
  constraint coincident L39 P1
  constraint coincident L38.end L36
  constraint coincident L38.end L35
  constraint tangent L36 A20
  constraint tangent L35 A20
  constraint coincident L39.end L37
  constraint coincident L39.end L36
  constraint tangent L37 A21
  constraint tangent L36 A21
  constraint coincident L39.start L35
  constraint coincident L39.start L34
  constraint tangent L35 A22
  constraint tangent L34 A22
  constraint coincident L38.start L37
  constraint coincident L38.start L34
  constraint tangent L37 A23
  constraint tangent L34 A23
  constraint horizontal L40
  constraint perpendicular L40 L41
  constraint parallel L40 L42
  constraint parallel L41 L43
  constraint coincident L44 P2
  constraint coincident L45 P2
  constraint horizontal L46
  constraint perpendicular L46 L47
  constraint parallel L46 L48
  constraint parallel L47 L49
  constraint midpoint L2 L50.start
  constraint midpoint L6 L50.end
  measures "d1" distance of L1.end L2.end
  measures "d2" distance of L0.end L1.end
  measures "d4" diameter of A0
  measures "d5" distance of L7 P0
  measures "d6" distance of L8 P0
  measures "d7" diameter of A1
  measures "d8" diameter of A2
  measures "d9" diameter of A3
  measures "d10" distance of L6 A1.centre
  measures "d11" distance of L7 A1.centre
  measures "d12" distance of L9 A2.centre
  measures "d13" distance of L8 A2.centre
  measures "d14" distance of L0 A3.centre
  measures "d15" distance of L9 A3.centre
  measures "d18" distance of L7.end L8.end
  measures "d37" distance of L21 L24
  measures "d38" distance of L11 L25
  measures "d39" distance of L10 L26
  measures "d40" distance of L18 L27
  measures "d41" distance of L20 L30
  measures "d42" distance of L12 L31
  measures "d43" distance of L19 L32
  measures "d44" distance of L22 L33
  measures "d71" distance of L38.end L39.end
  measures "d72" distance of L39.start L38.end
  measures "d73" radius of A20
  measures "d74" radius of A21
  measures "d75" radius of A22
  measures "d76" radius of A23
  measures "d79" distance of L24.end L24.start
  measures "d80" distance of L41.end L42.end
  measures "d81" distance of L40.end L41.end
  measures "d82" distance of L22 P2
  measures "d83" distance of L21 P2
  measures "d84" distance of L47.end L40.end
  measures "d85" distance of L46.end L47.end
  measures "d86" distance of L25 L35
  measures "d87" distance of L24 L36
extrude "Extrude1" add sketch "Main" along normal blind 10 contours L0 L1 L2 L3 | L6 L7 L8 L9 | A4 A5 L10 A6 L11 A7 L12 L29 | L13 A8 L14 A9 L15 A10 A11 L16 | L17 A12 L18 A13 L19 A14 A15 L28 | A16 A17 L20 A18 L21 A19 L22 L23 | L24 L25 L30 L31 | L24 L25 L26 L27 L30 L31 L32 L33 | L24 L27 L32 L33 | L34 L35 L36 L37 A20 A21 A22 A23 | L46 L47 L48 L49 | L40 L41 L42 L43 | A24 L51 A25 L52 A26 L53 A27 L54 | S0 S1 S2 S3 S4 S5 S6 S7 S8 S9 S10 S11 S12 S13 S14 S15 S16 S17 S18 S19 S20 S21 S22 S23 S24 S25 S26 S27 S28 S29 S30 S31 S32 S33 S34 S35 S36 S37 S38 S39 S40 S41 S42 S43 S44 S45 S46 S47 S48 S49 S50 S51 S52 S53 S54 S55 S56 S57 S58 S59 S60 S61 S62 S63 S64 S65 S66 S67 S68 S69 S70 S71 S72 S73 S74 S75 S76 S77 S78 S79 S80 S81 S82 S83 S84 S85 S86 S87 S88 S89 S90 S91 S92 S93 S94 S95 S96 S97 S98 S99 S100 S101 S102 S103 S104 S105 S106 S107 S108 S109 S110 S111 S112 S113 S114 S115 S116 S117 S118 S119 S120 S121 S122 S123 S124 | S125 S126 S127 S128 S129 S130 S131 S132 S153 S154 S155 S156 S157 S158 S159 S160 | S133 S134 S135 S136 S137 S138 S139 S161 S162 S163 S164 S165 S166 S167 | S140 S141 S142 S143 S144 S145 S146 S147 S148 S149 S150 S151 S152 S168 S169 S170 S171 S172 S173 S174 S175 S176 S177 S178 S179 S180 makes body 1
sketch "Side" plane through (43.9, 0, 0) normal (1, 0, 0) x (0, 1, 0)
  line L0 (-33.9, 0) -> (33.9, 0)
  line L1 (33.9, 0) -> (33.9, 10)
  line L2 (33.9, 10) -> (-33.9, 10)
  line L3 (-33.9, 10) -> (-33.9, 0)
  line L4 (33.9, 0) -> (-33.9, 5)
  constraint coincident L0.end L1.start
  constraint midpoint L3 L4.end
extrude "Extrude2" cut sketch "Side" against normal blind 87.8 contours L0 L3 L4 bodies 1
extrude "Extrude4" add sketch "Main" along normal blind 9.6 from surface at 10 contours L6 L7 L8 L9 bodies 1
extrude "Extrude5" add sketch "Main" along normal blind 3 from surface at 19.6 separate body contours L0 L1 L2 L3 | L6 L7 L8 L9 | L24 L25 L30 L31 | L24 L25 L26 L27 L30 L31 L32 L33 | L24 L27 L32 L33 | L46 L47 L48 L49 | L40 L41 L42 L43 | A24 L51 A25 L52 A26 L53 A27 L54 | S0 S1 S2 S3 S4 S5 S6 S7 S8 S9 S10 S11 S12 S13 S14 S15 S16 S17 S18 S19 S20 S21 S22 S23 S24 S25 S26 S27 S28 S29 S30 S31 S32 S33 S34 S35 S36 S37 S38 S39 S40 S41 S42 S43 S44 S45 S46 S47 S48 S49 S50 S51 S52 S53 S54 S55 S56 S57 S58 S59 S60 S61 S62 S63 S64 S65 S66 S67 S68 S69 S70 S71 S72 S73 S74 S75 S76 S77 S78 S79 S80 S81 S82 S83 S84 S85 S86 S87 S88 S89 S90 S91 S92 S93 S94 S95 S96 S97 S98 S99 S100 S101 S102 S103 S104 S105 S106 S107 S108 S109 S110 S111 S112 S113 S114 S115 S116 S117 S118 S119 S120 S121 S122 S123 S124 | S125 S126 S127 S128 S129 S130 S131 S132 S153 S154 S155 S156 S157 S158 S159 S160 | S133 S134 S135 S136 S137 S138 S139 S161 S162 S163 S164 S165 S166 S167 | S140 S141 S142 S143 S144 S145 S146 S147 S148 S149 S150 S151 S152 S168 S169 S170 S171 S172 S173 S174 S175 S176 S177 S178 S179 S180 makes body 2
extrude "Extrude6" add sketch "Main" along normal blind 3 from surface at 22.6 separate body contours L0 L1 L2 L3 | L6 L7 L8 L9 | L24 L25 L30 L31 | L24 L27 L32 L33 | A24 L51 A25 L52 A26 L53 A27 L54 | S0 S1 S2 S3 S4 S5 S6 S7 S8 S9 S10 S11 S12 S13 S14 S15 S16 S17 S18 S19 S20 S21 S22 S23 S24 S25 S26 S27 S28 S29 S30 S31 S32 S33 S34 S35 S36 S37 S38 S39 S40 S41 S42 S43 S44 S45 S46 S47 S48 S49 S50 S51 S52 S53 S54 S55 S56 S57 S58 S59 S60 S61 S62 S63 S64 S65 S66 S67 S68 S69 S70 S71 S72 S73 S74 S75 S76 S77 S78 S79 S80 S81 S82 S83 S84 S85 S86 S87 S88 S89 S90 S91 S92 S93 S94 S95 S96 S97 S98 S99 S100 S101 S102 S103 S104 S105 S106 S107 S108 S109 S110 S111 S112 S113 S114 S115 S116 S117 S118 S119 S120 S121 S122 S123 S124 | S125 S126 S127 S128 S129 S130 S131 S132 S153 S154 S155 S156 S157 S158 S159 S160 | S133 S134 S135 S136 S137 S138 S139 S161 S162 S163 S164 S165 S166 S167 | S140 S141 S142 S143 S144 S145 S146 S147 S148 S149 S150 S151 S152 S168 S169 S170 S171 S172 S173 S174 S175 S176 S177 S178 S179 S180 makes body 3
fillet "Fillet2" radius 3 8 edges at (-21.65, 2.525, 25.6) (-31.175, -9.525, 25.6) (-0.075, -21.575, 25.6) (-0.075, 21.575, 25.6) (-12.125, 12.05, 25.6) (11.975, 12.05, 25.6) (21.5, 2.525, 25.6) (31.025, -9.525, 25.6) on bodies 3
fillet "Fillet3" radius 5 16 edges at (-43.9, -33.9, 7.5) (43.9, -33.9, 7.5) (-43.9, 33.9, 5) (43.9, 33.9, 5) (-43.9, -33.9, 12.3) (43.9, -33.9, 12.3) (-43.9, 33.9, 9.8) (43.9, 33.9, 9.8) (-43.9, -33.9, 21.1) (43.9, -33.9, 21.1) (-43.9, 33.9, 21.1) (43.9, 33.9, 21.1) (-43.9, -33.9, 24.1) (43.9, -33.9, 24.1) (-43.9, 33.9, 24.1) (43.9, 33.9, 24.1) on bodies 1 2 3
chamfer "Chamfer3" distance 2 angle 45 8 edges at (0, -33.9, 25.6) (42.4355, -32.4355, 25.6) (43.9, 0, 25.6) (42.4355, 32.4355, 25.6) (0, 33.9, 25.6) (-42.4355, 32.4355, 25.6) (-43.9, 0, 25.6) (-42.4355, -32.4355, 25.6) on bodies 3
sketch "USB" plane through (0, 23.9, 0) normal (0, -1, 0) x (1, 0, 0)
  line L0 (33.9, 10) -> (33.9, 19.6)
  line L1 (33.9, 19.6) -> (-33.9, 19.6)
  line L2 (-33.9, 19.6) -> (-33.9, 10)
  line L3 (15.9, 18.55) -> (25.9, 18.55)
  line L4 (26.9, 17.55) -> (26.9, 12.05)
  line L5 (25.9, 11.05) -> (15.9, 11.05)
  line L6 (14.9, 12.05) -> (14.9, 17.55)
  arc A0 (26.9, 17.55) -> (25.9, 18.55) centre (25.9, 17.55) ccw
  arc A1 (15.9, 18.55) -> (14.9, 17.55) centre (15.9, 17.55) ccw
  arc A2 (14.9, 12.05) -> (15.9, 11.05) centre (15.9, 12.05) ccw
  arc A3 (25.9, 11.05) -> (26.9, 12.05) centre (25.9, 12.05) ccw
  line L7 (-33.9, 10) -> (33.9, 10)
  point P0 (14.9, 18.55)
  point P1 (26.9, 18.55)
  dimension "d54" = 7
  dimension "d55" = 12
  dimension "d56" = 1
  dimension "d57" = 7.5
  dimension "d65" = 1.05
  constraint horizontal L3
  constraint vertical L4
  constraint horizontal L5
  constraint vertical L6
  constraint coincident P1 L3
  constraint coincident P1 L4
  constraint tangent L3 A0
  constraint tangent L4 A0
  constraint coincident P0 L3
  constraint coincident P0 L6
  constraint tangent L3 A1
  constraint tangent L6 A1
  constraint equal A0 A1
  constraint tangent L5 A2
  constraint tangent L6 A2
  constraint equal A0 A2
  constraint tangent L5 A3
  constraint tangent L4 A3
  constraint equal A0 A3
  measures "d54" distance of L0 L4
  measures "d55" distance of P0 P1
  measures "d56" radius of A0
  measures "d57" distance of L3 L5
  measures "d65" distance of L1 L3
extrude "Extrude7" cut sketch "USB" against normal blind 25 contours L3 L4 L5 L6 A0 A1 A2 A3 bodies 1
fillet "Fillet4" radius 5 8 edges at (26.9, 33.9, 14.8) (26.6071, 33.9, 18.2571) (20.9, 33.9, 18.55) (15.1929, 33.9, 18.2571) (14.9, 33.9, 14.8) (15.1929, 33.9, 11.3429) (20.9, 33.9, 11.05) (26.6071, 33.9, 11.3429) on bodies 1
extrude "Extrude8" add sketch "Main" along normal blind 1.6 from surface at 17 separate body contours L0 L1 L2 L3 | A4 A5 L10 A6 L11 A7 L12 L29 | L13 A8 L14 A9 L15 A10 A11 L16 | L17 A12 L18 A13 L19 A14 A15 L28 | A16 A17 L20 A18 L21 A19 L22 L23 | L24 L25 L30 L31 | L24 L25 L26 L27 L30 L31 L32 L33 | L24 L27 L32 L33 | L34 L35 L36 L37 A20 A21 A22 A23 | L46 L47 L48 L49 | L40 L41 L42 L43 | A24 L51 A25 L52 A26 L53 A27 L54 | S0 S1 S2 S3 S4 S5 S6 S7 S8 S9 S10 S11 S12 S13 S14 S15 S16 S17 S18 S19 S20 S21 S22 S23 S24 S25 S26 S27 S28 S29 S30 S31 S32 S33 S34 S35 S36 S37 S38 S39 S40 S41 S42 S43 S44 S45 S46 S47 S48 S49 S50 S51 S52 S53 S54 S55 S56 S57 S58 S59 S60 S61 S62 S63 S64 S65 S66 S67 S68 S69 S70 S71 S72 S73 S74 S75 S76 S77 S78 S79 S80 S81 S82 S83 S84 S85 S86 S87 S88 S89 S90 S91 S92 S93 S94 S95 S96 S97 S98 S99 S100 S101 S102 S103 S104 S105 S106 S107 S108 S109 S110 S111 S112 S113 S114 S115 S116 S117 S118 S119 S120 S121 S122 S123 S124 | S125 S126 S127 S128 S129 S130 S131 S132 S153 S154 S155 S156 S157 S158 S159 S160 | S133 S134 S135 S136 S137 S138 S139 S161 S162 S163 S164 S165 S166 S167 | S140 S141 S142 S143 S144 S145 S146 S147 S148 S149 S150 S151 S152 S168 S169 S170 S171 S172 S173 S174 S175 S176 S177 S178 S179 S180 makes body 4
fillet "Fillet5" radius 1.5 4 edges at (-33.9, -23.9, 17.8) (33.9, -23.9, 17.8) (-33.9, 23.9, 17.8) (33.9, 23.9, 17.8) on bodies 4
extrude "Extrude9" cut sketch "Main" along normal blind 1 from surface at 24.6 contours S0 S1 S2 S3 S4 S5 S6 S7 S8 S9 S10 S11 S12 S13 S14 S15 S16 S17 S18 S19 S20 S21 S22 S23 S24 S25 S26 S27 S28 S29 S30 S31 S32 S33 S34 S35 S36 S37 S38 S39 S40 S41 S42 S43 S44 S45 S46 S47 S48 S49 S50 S51 S52 S53 S54 S55 S56 S57 S58 S59 S60 S61 S62 S63 S64 S65 S66 S67 S68 S69 S70 S71 S72 S73 S74 S75 S76 S77 S78 S79 S80 S81 S82 S83 S84 S85 S86 S87 S88 S89 S90 S91 S92 S93 S94 S95 S96 S97 S98 S99 S100 S101 S102 S103 S104 S105 S106 S107 S108 S109 S110 S111 S112 S113 S114 S115 S116 S117 S118 S119 S120 S121 S122 S123 S124 bodies 3
named bodies: "Base", "Plate", "Shell", "PCB"
